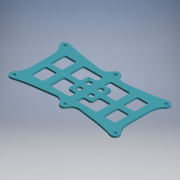
# Autodesk Inventor part: Body_bottom
Saved by Autodesk Inventor 2017 (Build 210142000, 142)
## iProperties
Part Number: Body_bottom
Material: Generic
Document SubType Name: Modeling
Designer: alex-
Appearance: Cadet Blue
b_mat_thickness: 0,500 cm
b_core_width: 15,000 cm
b_leg_space: 15,000 cm
Author: alex-
Autodesk Inventor part; units mm, degrees
ref_plane "YZ Plane" through (0, 0, 0) normal (1, 0, 0) x (0, 1, 0)
ref_plane "XZ Plane" through (0, 0, 0) normal (0, 1, 0) x (-1, 0, 0)
ref_plane "XY Plane" through (0, 0, 0) normal (0, 0, 1) x (1, 0, 0)
sketch "Sketch1" plane through (0, 0, 0) normal (0, 1, 0) x (-1, 0, 0)
  line L0 (166.0997, -69.6334) -> (155.3666, -91.0997)
  line L1 (155.3666, -91.0997) -> (133.9003, -80.3666)
  line L2 (133.9003, -80.3666) -> (144.6334, -58.9003) construction
  line L3 (144.6334, -58.9003) -> (166.0997, -69.6334)
  line L4 (144.6334, -58.9003) -> (155.3666, -91.0997) construction
  line L5 (12, -87) -> (-12, -87)
  line L6 (-12, -87) -> (-12, -63)
  line L7 (-12, -63) -> (12, -63) construction
  line L8 (12, -63) -> (12, -87)
  line L9 (12, -63) -> (-12, -87) construction
  line L10 (-155.3666, -91.0997) -> (-166.0997, -69.6334)
  line L11 (-166.0997, -69.6334) -> (-144.6334, -58.9003)
  line L12 (-144.6334, -58.9003) -> (-133.9003, -80.3666) construction
  line L13 (-133.9003, -80.3666) -> (-155.3666, -91.0997)
  line L14 (-133.9003, -80.3666) -> (-166.0997, -69.6334) construction
  line L15 (155.3666, 91.0997) -> (166.0997, 69.6334)
  line L16 (166.0997, 69.6334) -> (144.6334, 58.9003)
  line L17 (144.6334, 58.9003) -> (133.9003, 80.3666) construction
  line L18 (133.9003, 80.3666) -> (155.3666, 91.0997)
  line L19 (133.9003, 80.3666) -> (166.0997, 69.6334) construction
  line L20 (12, 63) -> (-12, 63) construction
  line L21 (-12, 63) -> (-12, 87)
  line L22 (-12, 87) -> (12, 87)
  line L23 (12, 87) -> (12, 63)
  line L24 (12, 87) -> (-12, 63) construction
  line L25 (-166.0997, 69.6334) -> (-155.3666, 91.0997)
  line L26 (-155.3666, 91.0997) -> (-133.9003, 80.3666)
  line L27 (-133.9003, 80.3666) -> (-144.6334, 58.9003) construction
  line L28 (-144.6334, 58.9003) -> (-166.0997, 69.6334)
  line L29 (-144.6334, 58.9003) -> (-155.3666, 91.0997) construction
  line L30 (160.7331, -80.3666) -> (-160.7331, -80.3666) construction
  line L31 (-160.7331, -80.3666) -> (-160.7331, 80.3666) construction
  line L32 (-160.7331, 80.3666) -> (160.7331, 80.3666) construction
  line L33 (160.7331, 80.3666) -> (160.7331, -80.3666) construction
  line L34 (160.7331, -80.3666) -> (-160.7331, 80.3666) construction
  line L35 (160.7331, 80.3666) -> (-160.7331, -80.3666) construction
  line L36 (133.9003, 80.3666) -> (12, 63)
  line L37 (-12, 63) -> (-133.9003, 80.3666)
  line L38 (-144.6334, 58.9003) -> (-144.6334, -58.9003)
  line L39 (-133.9003, -80.3666) -> (-12, -63)
  line L40 (12, -63) -> (133.9003, -80.3666)
  line L41 (144.6334, -58.9003) -> (144.6334, 58.9003)
  point P0 (0, 0)
  point P1 (0, 0)
  point P2 (144.6334, -85.7331)
  point P3 (144.6334, 85.7331)
  point P4 (0, 0)
  point P5 (0, -75)
  point P6 (150, -75)
  point P7 (0, 75)
  point P8 (150, 75)
  point P9 (-150, 75)
  dimension "d27" = 24
  dimension "d28" = 24
  dimension "d30" = 24
  dimension "d32" = 24
  dimension "d34" = 24
  dimension "d36" = 24
  dimension "d40" = 150
  dimension "d42" = 150
  constraints: 84 end point, 17 perpendicular, 15 parallel, 13 midpoint, 2 horizontal, 2 horizontal alignment, 2 vertical alignment, 1 coincident, 1 point on line
  measures "d27" distance of L0.start L0.end
  measures "d28" distance of L5.start L5.end
  measures "d30" distance of L10.start L10.end
  measures "d32" distance of L15.start L15.end
  measures "d34" distance of L20.start L20.end
  measures "d36" distance of L25.start L25.end
  measures "d40" distance of point (150, -75) point (150, 75)
  measures "d42" distance of point (0, 75) point (150, 75)
extrude "Extrusion1" add sketch "Sketch1" along normal blind 5
fillet "Fillet3" radius 12 12 edges at (-155.3666, 2.5, 91.0997) (-166.0997, 2.5, 69.6334) (-166.0997, 2.5, -69.6334) (-155.3666, 2.5, -91.0997) (-12, 2.5, -87) (12, 2.5, -87) (155.3666, 2.5, -91.0997) (166.0997, 2.5, -69.6334) (166.0997, 2.5, 69.6334) (155.3666, 2.5, 91.0997) (12, 2.5, 87) (-12, 2.5, 87)
fillet "Fillet4" radius 24 4 edges at (-12, 2.5, 63) (12, 2.5, 63) (-12, 2.5, -63) (12, 2.5, -63)
fillet "Fillet5" radius 360 4 edges at (-133.9003, 2.5, 80.3666) (133.9003, 2.5, 80.3666) (133.9003, 2.5, -80.3666) (-133.9003, 2.5, -80.3666)
fillet "Fillet6" radius 48 4 edges at (-144.6334, 2.5, 58.9003) (-144.6334, 2.5, -58.9003) (144.6334, 2.5, -58.9003) (144.6334, 2.5, 58.9003)
sketch "Sketch5" plane through (0, 5, 0) normal (0, 1, 0) x (1, 0, 0)
  line L0 (-124.6334, 50) -> (124.6334, 50)
  line L1 (124.6334, 50) -> (124.6334, -50)
  line L2 (124.6334, -50) -> (-124.6334, -50)
  line L3 (-124.6334, -50) -> (-124.6334, 50)
  line L4 (-144.6334, 32.7816) -> (-144.6334, -32.7816) construction
  arc A0 (10.8805, 80.061) -> (-10.8805, 80.061) centre (0, 75) ccw construction
  line L5 (-35, 30.75) -> (35, 30.75)
  line L6 (35, 30.75) -> (35, -30.75)
  line L7 (35, -30.75) -> (-35, -30.75)
  line L8 (-35, -30.75) -> (-35, 30.75)
  line L9 (-25, 20.75) -> (25, 20.75)
  line L10 (25, 20.75) -> (25, -20.75)
  line L11 (25, -20.75) -> (-25, -20.75)
  line L12 (-25, -20.75) -> (-25, 20.75)
  line L13 (-25, 7.5) -> (-10, 7.5)
  line L14 (-10, 7.5) -> (-10, 20.75)
  line L15 (10, 20.75) -> (10, 7.5)
  line L16 (10, 7.5) -> (25, 7.5)
  line L17 (25, -7.5) -> (10, -7.5)
  line L18 (10, -7.5) -> (10, -20.75)
  line L19 (-25, -7.5) -> (-10, -7.5)
  line L20 (-10, -7.5) -> (-10, -20.75)
  line L21 (-35, -7.5) -> (-124.6334, -7.5)
  line L22 (-35, 7.5) -> (-124.6334, 7.5)
  line L23 (35, 7.5) -> (124.6334, 7.5)
  line L24 (35, -7.5) -> (124.6334, -7.5)
  line L25 (-226.8, 0) -> (226.8, 0) construction
  line L26 (0, 121.8) -> (0, -121.8) construction
  line L27 (-10, 30.75) -> (-10, 50)
  line L28 (10, 30.75) -> (10, 50)
  line L29 (-10, -30.75) -> (-10, -50)
  line L30 (10, -30.75) -> (10, -50)
  line L31 (-89.8167, 50) -> (-89.8167, 7.5)
  line L32 (-69.8167, 50) -> (-69.8167, 7.5)
  line L33 (-89.8167, -7.5) -> (-89.8167, -50)
  line L34 (-69.8167, -7.5) -> (-69.8167, -50)
  line L35 (69.8167, 50) -> (69.8167, 7.5)
  line L36 (89.8167, 50) -> (89.8167, 7.5)
  line L37 (69.8167, -7.5) -> (69.8167, -50)
  line L38 (89.8167, -7.5) -> (89.8167, -50)
  line L39 (-89.8167, 28.75) -> (-69.8167, 28.75) construction
  line L40 (-79.8167, 28.75) -> (-79.8167, 20) construction
  circle A1 centre (-29, 24.5) radius 1.375
  circle A2 centre (29, 24.5) radius 1.375
  circle A3 centre (-29, -24.5) radius 1.375
  circle A4 centre (29, -24.5) radius 1.375
  point P0 (0, 0)
  point P1 (0, 50)
  point P2 (-124.6334, 0)
  point P3 (0, 30.75)
  point P4 (35, 0)
  point P5 (0, 20.75)
  point P6 (-25, 0)
  point P7 (1.6129, 86.8911)
  point P8 (-1.6129, 86.8911)
  dimension "d47" = 20
  dimension "d48" = 25
  dimension "d49" = 70
  dimension "d50" = 61.5
  dimension "d51" = 10
  dimension "d52" = 10
  dimension "d53" = 15
  dimension "d54" = 20
  dimension "d55" = 20
  dimension "d56" = 20
  dimension "d65" = 2.75
  dimension "d66" = 29
  dimension "d67" = 24.5
  constraints: 74 end point, 54 point on line, 11 parallel, 11 perpendicular, 10 horizontal alignment, 8 midpoint, 6 vertical alignment, 4 centre point, 3 horizontal, 3 symmetric about line, 3 vertical, 17 other
  measures "d47" distance between parallel lines of L4 L3
  measures "d49" distance of L5.start L5.end
  measures "d50" distance of L5.end L6.end
  measures "d51" distance between parallel lines of L8 L12
  measures "d52" distance between parallel lines of L5 L9
  measures "d53" distance between parallel lines of L23 L24
  measures "d54" distance between parallel lines of L28 L27
  measures "d55" distance between parallel lines of L32 L31
  measures "d56" distance between parallel lines of L36 L35
  measures "d65" diameter of A1
  measures "d66" distance from line of L26 A1.centre
  measures "d67" distance from line of L25 A1.centre
extrude "Extrusion3" cut sketch "Sketch5" against normal up to surface (5 mm away) contours L0 L31 L22 L3 | L0 L27 L5 L8 L22 L32 | L21 L33 L2 L3 | L0 L35 L23 L6 L5 L28 | L21 L8 L7 L29 L2 L34 | L0 L1 L23 L36 | L30 L7 L6 L24 L37 L2 | L1 L2 L38 L24 | L9 L14 L13 L12 | L9 L10 L16 L15 | L19 L20 L11 L12 | L10 L11 L18 L17 | A1 | A2 | A3 | A4
fillet "Fillet7" radius 5 56 edges at (-124.6334, 2.5, -50) (-89.8167, 2.5, -50) (-89.8167, 2.5, -7.5) (-124.6334, 2.5, -7.5) (-124.6334, 2.5, 7.5) (-89.8167, 2.5, 7.5) (-124.6334, 2.5, 50) (-89.8167, 2.5, 50) (-69.8167, 2.5, 50) (-69.8167, 2.5, 7.5) (-35, 2.5, 7.5) (-35, 2.5, 30.75) (-10, 2.5, 30.75) (-10, 2.5, 50) (-10, 2.5, 20.75) (-10, 2.5, 7.5) (-25, 2.5, 7.5) (-25, 2.5, 20.75) (-25, 2.5, -20.75) (-25, 2.5, -7.5) (-10, 2.5, -7.5) (-10, 2.5, -20.75) (10, 2.5, -20.75) (10, 2.5, -7.5) (25, 2.5, -7.5) (25, 2.5, -20.75) (-10, 2.5, -30.75) (-10, 2.5, -50) (-69.8167, 2.5, -50) (-69.8167, 2.5, -7.5) (-35, 2.5, -7.5) (10, 2.5, 7.5) (10, 2.5, 20.75) (25, 2.5, 20.75) (25, 2.5, 7.5) (10, 2.5, -50) (10, 2.5, -30.75) (69.8167, 2.5, -50) (35, 2.5, -30.75) (35, 2.5, -7.5) (69.8167, 2.5, -7.5) (89.8167, 2.5, -50) (124.6334, 2.5, -50) (124.6334, 2.5, -7.5) (89.8167, 2.5, -7.5) (89.8167, 2.5, 7.5) (124.6334, 2.5, 7.5) (124.6334, 2.5, 50) (89.8167, 2.5, 50) (35, 2.5, 7.5) (69.8167, 2.5, 7.5) (69.8167, 2.5, 50) (10, 2.5, 50) (10, 2.5, 30.75) (35, 2.5, 30.75) (-35, 2.5, -30.75)
sketch "Sketch6" plane through (0, 5, 0) normal (0, 1, 0) x (1, 0, 0)
  circle A0 centre (-150, 75) radius 3.75
  circle A1 centre (0, 75) radius 3.75
  circle A2 centre (150, 75) radius 3.75
  circle A3 centre (150, -75) radius 3.75
  circle A4 centre (0, -75) radius 3.75
  circle A5 centre (-150, -75) radius 3.75
  arc A6 (-146.5024, 86.479) -> (-158.5267, 66.5563) centre (-150, 75) ccw projected
  arc A7 (10.8805, 80.061) -> (-10.8805, 80.061) centre (0, 75) ccw projected
  arc A8 (158.5267, 66.5563) -> (146.5024, 86.479) centre (150, 75) ccw projected
  arc A9 (146.5024, -86.479) -> (158.5267, -66.5563) centre (150, -75) ccw projected
  arc A10 (-10.8805, -80.061) -> (10.8805, -80.061) centre (0, -75) ccw projected
  arc A11 (-158.5267, -66.5563) -> (-146.5024, -86.479) centre (-150, -75) ccw projected
  point P0 (0, 0)
  point P1 (1.6129, 86.8911)
  point P2 (-1.6129, 86.8911)
  point P3 (-1.6129, -86.8911)
  point P4 (1.6129, -86.8911)
  dimension "d60" = 7.5
  constraints: 6 centre point, 6 concentric, 5 equal radius
  measures "d60" diameter of A0
extrude "Extrusion4" cut sketch "Sketch6" against normal up to next
sketch "Sketch9" plane through (0, 5, 0) normal (0, 1, 0) x (1, 0, 0)
  circle A0 centre (-150, -75) radius 3.75 construction
  circle A1 centre (150, -75) radius 3.75 construction
  line L0 (-150, -75) -> (150, -75) construction
  circle A2 centre (-150, 75) radius 3.75 construction
  circle A3 centre (150, 75) radius 3.75 construction
  line L1 (-150, 75) -> (150, 75) construction
  circle A4 centre (-157, -75) radius 1
  circle A5 centre (-143, -75) radius 1
  circle A6 centre (-7, -75) radius 1
  circle A7 centre (7, -75) radius 1
  circle A8 centre (0, -75) radius 3.75 construction
  circle A9 centre (0, 75) radius 3.75 construction
  circle A10 centre (143, -75) radius 1
  circle A11 centre (157, -75) radius 1
  circle A12 centre (-157, 75) radius 1
  circle A13 centre (-143, 75) radius 1
  circle A14 centre (-7, 75) radius 1
  circle A15 centre (7, 75) radius 1
  circle A16 centre (143, 75) radius 1
  circle A17 centre (157, 75) radius 1
  point P0 (0, 0)
  dimension "d77" = 7
  dimension "d78" = 7
  dimension "d79" = 2
  dimension "d80" = 7
  dimension "d81" = 7
  dimension "d82" = 7
  dimension "d83" = 7
  dimension "d84" = 7
  dimension "d85" = 7
  dimension "d86" = 7
  dimension "d87" = 7
  dimension "d88" = 7
  dimension "d89" = 7
  constraints: 12 centre point, 11 equal radius, 7 point on line, 5 horizontal alignment, 4 end point, 2 horizontal
  measures "d77" distance of A4.centre L0.start
  measures "d78" distance of L0.start A5.centre
  measures "d79" diameter of A4
  measures "d80" distance of A6.centre A8.centre
  measures "d81" distance of A8.centre A7.centre
  measures "d82" distance of L0.end A10.centre
  measures "d83" distance of L0.end A11.centre
  measures "d84" distance of L1.start A12.centre
  measures "d85" distance of L1.start A13.centre
  measures "d86" distance of A9.centre A14.centre
  measures "d87" distance of A9.centre A15.centre
  measures "d88" distance of L1.end A16.centre
  measures "d89" distance of L1.end A17.centre
extrude "Extrusion6" cut sketch "Sketch9" against normal up to next
equation "\"d27\" = sa_diameter"
equation "\"d28\" = d29"
equation "\"d30\" = d31"
equation "\"d32\" = d33"
equation "\"d34\" = d35"
equation "\"d36\" = d37"
equation "\"d6\" = b_mat_thickness"
equation "\"b_mat_thickness\" = 5"
equation "\"b_core_width\" = 150"
equation "\"b_leg_space\" = 150"
equation "\"sa_diameter\" = 24"
equation "\"d29\" = 24"
equation "\"d31\" = 24"
equation "\"d33\" = 24"
equation "\"d35\" = 24"
equation "\"d37\" = 24"
body "Solid1"
